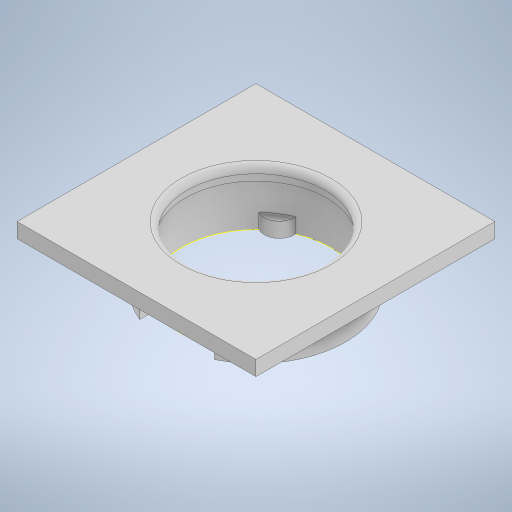
# Autodesk Inventor part: JoystickInsert
Saved by Autodesk Inventor 2024 (Build 280153000, 153)
## iProperties
Created: 2025-09-20
Part Number: JoystickInsert
Material: Generic
Document SubType Name: Modeling
Designer: Martin
Density: 1 g/cm^3
Appearance: Default
Author: Martin
Autodesk Inventor part; units mm, degrees
ref_plane "YZ Plane" through (0, 0, 0) normal (1, 0, 0) x (0, 1, 0)
sketch "Sketch1" plane through (0, 0, 0) normal (0, 1, 0) x (-1, 0, 0)
  line L0 (-25.4, 25.4) -> (25.4, 25.4)
  line L1 (25.4, 25.4) -> (25.4, -25.4)
  line L2 (25.4, -25.4) -> (-25.4, -25.4)
  line L3 (-25.4, -25.4) -> (-25.4, 25.4)
  line L4 (-25.4, 25.4) -> (25.4, -25.4) construction
  line L5 (25.4, 25.4) -> (-25.4, -25.4) construction
  point P0 (0, 0)
  dimension "d0" = 50.8
  dimension "d1" = 50.8
  constraints: 12 end point, 2 midpoint, 2 parallel, 1 horizontal, 1 perpendicular
  measures "d0" distance of L1.end L2.end
  measures "d1" distance of L0.end L1.end
extrude "Extrusion1" add sketch "Sketch1" along normal blind 3.1775
sketch "Sketch2" plane through (0, 0, 0) normal (0, -1, 0) x (1, 0, 0)
  circle A0 centre (0, 0) radius 15.875
  dimension "d4" = 31.75
  constraints: 1 centre point, 1 coincident
  measures "d4" diameter of A0
extrude "Extrusion2" cut sketch "Sketch2" against normal blind 3.1775
sketch "Sketch3" plane through (0, 0, 0) normal (0, -1, 0) x (1, 0, 0)
  circle A0 centre (0, 0) radius 19.05
  circle A1 centre (0, 0) radius 15.875 projected
  dimension "d7" = 38.1
  constraints: 1 centre point, 1 coincident
  measures "d7" diameter of A0
extrude "Extrusion3" add sketch "Sketch3" along normal blind 6.35
sketch "Sketch4" plane through (0, -6.35, 0) normal (0, -1, 0) x (1, 0, 0)
  circle A0 centre (0, 0) radius 19.05 projected
  line L0 (-9.35, 12.108) -> (11.15, 12.108) construction
  line L1 (11.15, 12.108) -> (11.15, -14.308) construction
  line L2 (11.15, -14.308) -> (-9.35, -14.308) construction
  line L3 (-9.35, -14.308) -> (-9.35, 12.108) construction
  circle A1 centre (11.15, -14.308) radius 1.016
  circle A2 centre (11.15, 12.108) radius 1.016
  circle A3 centre (-9.35, 12.108) radius 1.016
  circle A4 centre (-9.35, -14.308) radius 1.016
  circle A5 centre (0, 0) radius 15.875 projected
  circle A6 centre (0, 0) radius 19.05
  circle A7 centre (0, 0) radius 15.875
  circle A8 centre (11.15, -14.308) radius 3.175
  circle A9 centre (-9.35, -14.308) radius 3.175
  circle A10 centre (-9.35, 12.108) radius 3.175
  circle A11 centre (11.15, 12.108) radius 3.175
  line L4 (8.3095, 13.5265) -> (8.3095, 17.1422)
  line L5 (-7.0034, 14.2467) -> (-7.0034, 17.716)
  point P0 (11.15, -1.1)
  point P1 (0.9, 12.108)
  point P2 (14.0033, -12.9155)
  point P3 (-12.5247, -14.3539)
  point P4 (-8.1174, -17.234)
  point P5 (9.1025, -16.7346)
  point P6 (-12.0126, 10.3785)
  point P7 (-7.0034, 14.2467)
  point P8 (8.3095, 13.5265)
  point P9 (12.7973, 9.3938)
  point P10 (11.3128, -11.1372)
  point P11 (8.0355, -13.6911)
  point P12 (-6.1902, -14.6184)
  point P13 (-10.9029, -11.5387)
  dimension "d10" = 20.5
  dimension "d11" = 26.416
  dimension "d15" = 2.032
  dimension "d25" = 6.35
  dimension "d26" = 1.1
  dimension "d35" = 0.9
  constraints: 14 coincident, 12 end point, 8 centre point, 4 equal radius, 4 point on circle, 3 parallel, 2 concentric, 2 midpoint, 1 horizontal, 1 perpendicular, 1 vertical, 8 other
  measures "d10" distance of L1.end L2.end
  measures "d11" distance of L0.end L1.end
  measures "d15" diameter of A1
  measures "d25" diameter of A8
  measures "d26" vertical distance of point (0, 0) point (11.15, -1.1)
  measures "d35" horizontal distance of point (0.9, 12.108) A0.centre
ref_plane "Work Plane2" through (0, -9.525, 0) normal (0, -1, 0) x (1, 0, 0)
sketch "Sketch5" plane through (0, -9.525, 0) normal (0, -1, 0) x (1, 0, 0)
  circle A0 centre (0, 0) radius 15.875 projected
ref_plane "Work Plane1" through (0, 0, -25.4) normal (-1, 0, 0) x (0, 0, 1)
sketch "Sketch6" plane through (0, 0, -25.4) normal (-1, 0, 0) x (0, 0, 1)
  arc A0 (11.2224, 3.1775) -> (10.3522, 0) centre (25.4, -2.413) ccw
  line L0 (9.525, -6.35) -> (9.525, 3.1775) projected
  line L1 (9.525, 3.1775) -> (41.275, 3.1775) projected
  line L2 (44.45, 0) -> (6.35, 0) projected
  line L3 (11.2224, 3.1775) -> (9.525, 3.1775)
  line L4 (9.525, 3.1775) -> (9.525, 0)
  line L5 (9.525, 0) -> (10.3522, 0)
  line L6 (9.525, -9.525) -> (41.275, -9.525) projected
  line L7 (25.4, -2.413) -> (25.4, -9.525)
  point P0 (25.4, 0)
  point P1 (25.4, -5.969)
  dimension "d21" = 30.48
  dimension "d29" = 7.112
  constraints: 8 end point, 4 point on line, 2 midpoint, 2 point on circle, 1 centre point, 1 parallel, 1 vertical alignment
  measures "d21" diameter of A0
  measures "d29" distance of L7.start L7.end
revolve "Revolution1" add sketch "Sketch6" angle 360 about axis through (0, -2.413, 0) along (0, -1, 0)
fillet "Fillet1" radius 1.27 1 edges at (0, 3.1775, 14.1776)
extrude "Extrusion7" add sketch "Sketch4" along normal blind 3.175 contours A0 A11 L4 | L5 A10 A5 A9 A0 | A0 A11 A5 A2 | A5 A2 A11 | A9 A5 A0 | A0 A9 | A10 A5 A3 | A5 A3 A10 | A0 A8 A5 A11 | A9 A5 A8 A0 | A9 A5 | A8 A5 A0 A1 | A0 A1 A8 | A5 A8
sketch "Sketch7" plane through (0, -6.35, 0) normal (0, -1, 0) x (1, 0, 0)
  line L0 (-7.0034, 17.716) -> (-7.0034, 14.2467) projected
  arc A0 (8.3095, 13.5265) -> (-7.0034, 14.2467) centre (0, 0) ccw projected
  line L1 (8.3095, 13.5265) -> (8.3095, 17.1422) projected
  arc A1 (8.3095, 17.1422) -> (-7.0034, 17.716) centre (0, 0) ccw projected
extrude "Extrusion8" cut sketch "Sketch7" against normal blind 3.175
body "Solid1"
